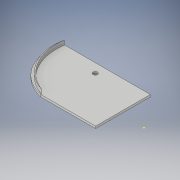
# Autodesk Inventor part: glassplane
Saved by Autodesk Inventor 2019 (Build 230136000, 136)
## iProperties
Created: 2020-02-20
Part Number: glassplane
Material: Generic
Document SubType Name: Modeling
Designer: ADMIN
Density: 1 g/cm^3
Appearance: Default
Author: ADMIN
Autodesk Inventor part; units mm, degrees
ref_plane "YZ Plane" through (0, 0, 0) normal (1, 0, 0) x (0, 1, 0)
ref_plane "XZ Plane" through (0, 0, 0) normal (0, 1, 0) x (-1, 0, 0)
ref_plane "XY Plane" through (0, 0, 0) normal (0, 0, 1) x (1, 0, 0)
sketch "Sketch1" plane through (0, 0, 0) normal (0, 1, 0) x (-1, 0, 0)
  point P0 (0, 0)
sketch "Sketch2" plane through (0, 0, 0) normal (0, 1, 0) x (-1, 0, 0)
  line L0 (506.9511, -135.755) -> (106.9511, -135.755)
  line L1 (106.9511, -135.755) -> (106.9511, 114.245)
  line L2 (106.9511, 114.245) -> (356.9511, 114.245)
  arc A0 (506.9511, -135.755) -> (356.9511, 114.245) centre (316.293, -80.1499) ccw
  point P0 (0, 0)
  dimension "d0" = 400
  dimension "d1" = 250
  dimension "d2" = 250
  constraints: 6 end point, 2 perpendicular, 2 point on circle, 1 centre point, 1 horizontal
  measures "d0" distance of L0.start L0.end
  measures "d1" distance of L0.end L1.end
  measures "d2" distance of L1.end L2.end
sketch "Sketch3" plane through (0, 0, 0) normal (0, 1, 0) x (-1, 0, 0)
  point P0 (0, 0)
extrude "Extrusion1" add sketch "Sketch2" along normal blind 10
sketch "Sketch4" plane through (0, 10, 0) normal (0, 1, 0) x (1, 0, 0)
  point P0 (0, 0)
  point P1 (-316.1297, 93.5657)
hole "Hole1" at (-316.1297, 10, -93.5657) direction (0, -1, 0) diameter 20 depth 8 tip angle 118
sketch "Sketch5" plane through (0, 10, 0) normal (0, 1, 0) x (1, 0, 0)
  arc A0 (-498.8992, 134.3673) -> (-354.956, -112.5228) centre (-289.3431, 91.1376) ccw
  arc A1 (-498.8992, 134.3673) -> (-354.956, -112.5228) centre (-271.7766, 101.3793) ccw
  point P0 (0, 0)
  constraints: 5 point on circle, 2 centre point
extrude "Extrusion2" add sketch "Sketch5" along normal blind 20
body "Solid1"
